Autodesk Fusion 360 part; units mm, degrees
(part 3 of 6)
  line L1808 (236.2761, -16.388) -> (236.2761, -22.338)
  line L1809 (236.2761, -22.338) -> (235.476, -22.338)
  line L1810 (235.476, -22.338) -> (235.476, -25.288)
  line L1811 (235.476, -25.288) -> (236.2761, -25.288)
  line L1812 (236.2761, -25.288) -> (236.2761, -26.288)
  line L1813 (236.2761, -26.288) -> (250.126, -26.288)
  line L1814 (250.126, -26.288) -> (250.126, -25.288)
  line L1815 (250.126, -25.288) -> (250.9261, -25.288)
  line L1816 (250.9261, -25.288) -> (250.9261, -22.338)
  line L1817 (250.9261, -22.338) -> (250.126, -22.338)
  line L1818 (250.126, -22.338) -> (250.126, -16.388)
  line L1819 (250.126, -16.388) -> (250.9261, -16.388)
  line L1820 (250.9261, -16.388) -> (250.9261, -13.438)
  line L1821 (250.9261, -13.438) -> (250.126, -13.438)
  line L1822 (250.126, -13.438) -> (250.126, -12.438)
  line L1823 (250.126, -12.438) -> (236.2761, -12.438)
  line L1824 (255.3261, -12.438) -> (255.3261, -13.438)
  line L1825 (255.3261, -13.438) -> (254.526, -13.438)
  line L1826 (254.526, -13.438) -> (254.526, -16.388)
  line L1827 (254.526, -16.388) -> (255.3261, -16.388)
  line L1828 (255.3261, -16.388) -> (255.3261, -22.338)
  line L1829 (255.3261, -22.338) -> (254.526, -22.338)
  line L1830 (254.526, -22.338) -> (254.526, -25.288)
  line L1831 (254.526, -25.288) -> (255.3261, -25.288)
  line L1832 (255.3261, -25.288) -> (255.3261, -26.288)
  line L1833 (255.3261, -26.288) -> (269.1765, -26.288)
  line L1834 (269.1765, -26.288) -> (269.1765, -25.288)
  line L1835 (269.1765, -25.288) -> (269.9755, -25.288)
  line L1836 (269.9755, -25.288) -> (269.9755, -22.338)
  line L1837 (269.9755, -22.338) -> (269.1765, -22.338)
  line L1838 (269.1765, -22.338) -> (269.1765, -16.388)
  line L1839 (269.1765, -16.388) -> (269.9755, -16.388)
  line L1840 (269.9755, -16.388) -> (269.9755, -13.438)
  line L1841 (269.9755, -13.438) -> (269.1765, -13.438)
  line L1842 (269.1765, -13.438) -> (269.1765, -12.438)
  line L1843 (269.1765, -12.438) -> (255.3261, -12.438)
extrude "Extrude1" add sketch "Sketch3" along normal blind 1.5 makes body 1
sketch "sketch 18250" plane through (138.5014, -57.3885, -4) normal (0, 0, 1) x (-1, 0, 0)
  line L0 (-186.1132, -52.3735) -> (-185.7375, -52.3875)
  line L1 (-185.7375, -52.3875) -> (128.5877, -52.3885)
  line L2 (128.5877, -52.3885) -> (128.9617, -52.3735)
  line L3 (128.9617, -52.3735) -> (129.3327, -52.3295)
  line L4 (129.3327, -52.3295) -> (129.6997, -52.2565)
  line L5 (129.6997, -52.2565) -> (130.0597, -52.1545)
  line L6 (130.0597, -52.1545) -> (130.4107, -52.0255)
  line L7 (130.4107, -52.0255) -> (130.7497, -51.8685)
  line L8 (130.7497, -51.8685) -> (131.0757, -51.6865)
  line L9 (131.0757, -51.6865) -> (131.3867, -51.4785)
  line L10 (131.3867, -51.4785) -> (131.6807, -51.2465)
  line L11 (131.6807, -51.2465) -> (131.9557, -50.9935)
  line L12 (131.9557, -50.9935) -> (132.2087, -50.7185)
  line L13 (132.2087, -50.7185) -> (132.4407, -50.4245)
  line L14 (132.4407, -50.4245) -> (132.6487, -50.1135)
  line L15 (132.6487, -50.1135) -> (132.8307, -49.7875)
  line L16 (132.8307, -49.7875) -> (132.9877, -49.4485)
  line L17 (132.9877, -49.4485) -> (133.1167, -49.0975)
  line L18 (133.1167, -49.0975) -> (133.2187, -48.7375)
  line L19 (133.2187, -48.7375) -> (133.2917, -48.3705)
  line L20 (133.2917, -48.3705) -> (133.3357, -47.9995)
  line L21 (133.3357, -47.9995) -> (133.3497, -47.6255)
  line L22 (133.3497, -47.6255) -> (133.3507, 76.2005)
  line L23 (133.3507, 76.2005) -> (133.3357, 76.5744)
  line L24 (133.3357, 76.5744) -> (133.2917, 76.9456)
  line L25 (133.2917, 76.9456) -> (133.2187, 77.3126)
  line L26 (133.2187, 77.3126) -> (133.1167, 77.6724)
  line L27 (133.1167, 77.6724) -> (132.9877, 78.0235)
  line L28 (132.9877, 78.0235) -> (132.8307, 78.3625)
  line L29 (132.8307, 78.3625) -> (132.6487, 78.6884)
  line L30 (132.6487, 78.6884) -> (132.4407, 78.9996)
  line L31 (132.4407, 78.9996) -> (132.2087, 79.2935)
  line L32 (132.2087, 79.2935) -> (131.9557, 79.5684)
  line L33 (131.9557, 79.5684) -> (131.6807, 79.8216)
  line L34 (131.6807, 79.8216) -> (131.3867, 80.0534)
  line L35 (131.3867, 80.0534) -> (131.0757, 80.2614)
  line L36 (131.0757, 80.2614) -> (130.7497, 80.4434)
  line L37 (130.7497, 80.4434) -> (130.4107, 80.6006)
  line L38 (130.4107, 80.6006) -> (130.0597, 80.7294)
  line L39 (130.0597, 80.7294) -> (129.6997, 80.8316)
  line L40 (129.6997, 80.8316) -> (129.3327, 80.9046)
  line L41 (129.3327, 80.9046) -> (128.9617, 80.9485)
  line L42 (128.9617, 80.9485) -> (128.5877, 80.9636)
  line L43 (128.5877, 80.9636) -> (-185.7375, 80.9636)
  line L44 (-185.7375, 80.9636) -> (-186.1132, 80.9485)
  line L45 (-186.1132, 80.9485) -> (-186.4836, 80.9046)
  line L46 (-186.4836, 80.9046) -> (-186.8514, 80.8316)
  line L47 (-186.8514, 80.8316) -> (-187.2112, 80.7294)
  line L48 (-187.2112, 80.7294) -> (-187.5605, 80.6006)
  line L49 (-187.5605, 80.6006) -> (-187.8992, 80.4434)
  line L50 (-187.8992, 80.4434) -> (-188.2272, 80.2614)
  line L51 (-188.2272, 80.2614) -> (-188.5368, 80.0534)
  line L52 (-188.5368, 80.0534) -> (-188.8305, 79.8216)
  line L53 (-188.8305, 79.8216) -> (-189.1057, 79.5684)
  line L54 (-189.1057, 79.5684) -> (-189.3597, 79.2935)
  line L55 (-189.3597, 79.2935) -> (-189.5925, 78.9996)
  line L56 (-189.5925, 78.9996) -> (-189.7989, 78.6884)
  line L57 (-189.7989, 78.6884) -> (-189.9814, 78.3625)
  line L58 (-189.9814, 78.3625) -> (-190.1375, 78.0235)
  line L59 (-190.1375, 78.0235) -> (-190.2672, 77.6724)
  line L60 (-190.2672, 77.6724) -> (-190.3704, 77.3126)
  line L61 (-190.3704, 77.3126) -> (-190.4418, 76.9456)
  line L62 (-190.4418, 76.9456) -> (-190.4868, 76.5744)
  line L63 (-190.4868, 76.5744) -> (-190.5, 76.2005)
  line L64 (-190.5, 76.2005) -> (-190.5, -47.6255)
  line L65 (-190.5, -47.6255) -> (-190.4868, -47.9995)
  line L66 (-190.4868, -47.9995) -> (-190.4418, -48.3705)
  line L67 (-190.4418, -48.3705) -> (-190.3704, -48.7375)
  line L68 (-190.3704, -48.7375) -> (-190.2672, -49.0975)
  line L69 (-190.2672, -49.0975) -> (-190.1375, -49.4485)
  line L70 (-190.1375, -49.4485) -> (-189.9814, -49.7875)
  line L71 (-189.9814, -49.7875) -> (-189.7989, -50.1135)
  line L72 (-189.7989, -50.1135) -> (-189.5925, -50.4245)
  line L73 (-189.5925, -50.4245) -> (-189.3597, -50.7185)
  line L74 (-189.3597, -50.7185) -> (-189.1057, -50.9935)
  line L75 (-189.1057, -50.9935) -> (-188.8305, -51.2465)
  line L76 (-188.8305, -51.2465) -> (-188.5368, -51.4785)
  line L77 (-188.5368, -51.4785) -> (-188.2272, -51.6865)
  line L78 (-188.2272, -51.6865) -> (-187.8992, -51.8685)
  line L79 (-187.8992, -51.8685) -> (-187.5605, -52.0255)
  line L80 (-187.5605, -52.0255) -> (-187.2112, -52.1545)
  line L81 (-187.2112, -52.1545) -> (-186.8514, -52.2565)
  line L82 (-186.8514, -52.2565) -> (-186.4836, -52.3295)
  line L83 (-186.4836, -52.3295) -> (-186.1132, -52.3735)
  circle A0 centre (128.5875, 76.2) radius 1.1
  arc A1 (117.7379, 65.4486) -> (118.4252, 66.1358) centre (117.9984, 65.8753) ccw
  arc A2 (117.7379, 65.4486) -> (117.5816, 65.4925) centre (117.5817, 65.1928) ccw
  line L84 (117.5816, 65.4925) -> (116.6813, 65.4925)
  line L85 (116.6813, 65.4925) -> (115.7809, 65.4925)
  arc A3 (115.7809, 65.4925) -> (115.6246, 65.4486) centre (115.7809, 65.1925) ccw
  arc A4 (114.9373, 66.1358) -> (115.6246, 65.4486) centre (115.3641, 65.8753) ccw
  arc A5 (114.9373, 66.1358) -> (114.9812, 66.2921) centre (114.6813, 66.2921) ccw
  line L86 (114.9812, 66.2921) -> (114.9813, 66.9925)
  line L87 (114.9813, 66.9925) -> (114.9813, 67.6929)
  arc A6 (114.9813, 67.6929) -> (114.9373, 67.8492) centre (114.6813, 67.6929) ccw
  arc A7 (115.6246, 68.5364) -> (114.9373, 67.8492) centre (115.3641, 68.1097) ccw
  arc A8 (115.6246, 68.5364) -> (115.7809, 68.4925) centre (115.7809, 68.7925) ccw
  line L88 (115.7809, 68.4925) -> (116.6813, 68.4925)
  line L89 (116.6813, 68.4925) -> (117.5816, 68.4925)
  arc A9 (117.5816, 68.4925) -> (117.7379, 68.5364) centre (117.5816, 68.7925) ccw
  arc A10 (118.4252, 67.8492) -> (117.7379, 68.5364) centre (117.9984, 68.1097) ccw
  arc A11 (118.4252, 67.8492) -> (118.3812, 67.6929) centre (118.6813, 67.6928) ccw
  line L90 (118.3812, 67.6929) -> (118.3812, 66.9925)
  line L91 (118.3812, 66.9925) -> (118.3812, 66.2921)
  arc A12 (118.3812, 66.2921) -> (118.4252, 66.1358) centre (118.6813, 66.2922) ccw
  circle A13 centre (121.7613, 61.9125) radius 0.875
  circle A14 centre (116.6813, 61.9125) radius 1.9939
  circle A15 centre (111.6013, 61.9125) radius 0.875
  arc A16 (93.9254, 65.4486) -> (94.6127, 66.1358) centre (94.1859, 65.8753) ccw
  arc A17 (93.9254, 65.4486) -> (93.7691, 65.4925) centre (93.7692, 65.1928) ccw
  line L92 (93.7691, 65.4925) -> (92.8688, 65.4925)
  line L93 (92.8688, 65.4925) -> (91.9684, 65.4925)
  arc A18 (91.9684, 65.4925) -> (91.8121, 65.4486) centre (91.9684, 65.1925) ccw
  arc A19 (91.1248, 66.1358) -> (91.8121, 65.4486) centre (91.5516, 65.8753) ccw
  arc A20 (91.1248, 66.1358) -> (91.1687, 66.2921) centre (90.8688, 66.2921) ccw
  line L94 (91.1687, 66.2921) -> (91.1688, 66.9925)
  line L95 (91.1688, 66.9925) -> (91.1688, 67.6929)
  arc A21 (91.1688, 67.6929) -> (91.1248, 67.8492) centre (90.8688, 67.6929) ccw
  arc A22 (91.8121, 68.5364) -> (91.1248, 67.8492) centre (91.5516, 68.1097) ccw
  arc A23 (91.8121, 68.5364) -> (91.9684, 68.4925) centre (91.9684, 68.7925) ccw
  line L96 (91.9684, 68.4925) -> (92.8688, 68.4925)
  line L97 (92.8688, 68.4925) -> (93.7691, 68.4925)
  arc A24 (93.7691, 68.4925) -> (93.9254, 68.5364) centre (93.7691, 68.7925) ccw
  arc A25 (94.6127, 67.8492) -> (93.9254, 68.5364) centre (94.1859, 68.1097) ccw
  arc A26 (94.6127, 67.8492) -> (94.5687, 67.6929) centre (94.8688, 67.6928) ccw
  line L98 (94.5687, 67.6929) -> (94.5687, 66.9925)
  line L99 (94.5687, 66.9925) -> (94.5687, 66.2921)
  arc A27 (94.5687, 66.2921) -> (94.6127, 66.1358) centre (94.8688, 66.2922) ccw
  circle A28 centre (97.9488, 61.9125) radius 0.875
  circle A29 centre (92.8688, 61.9125) radius 1.9939
  circle A30 centre (87.7887, 61.9125) radius 0.875
  circle A31 centre (74.1363, 61.9125) radius 0.875
  arc A32 (70.1129, 65.4486) -> (70.8002, 66.1358) centre (70.3734, 65.8753) ccw
  arc A33 (70.1129, 65.4486) -> (69.9566, 65.4925) centre (69.9567, 65.1928) ccw
  line L100 (69.9566, 65.4925) -> (69.0563, 65.4925)
  line L101 (69.0563, 65.4925) -> (68.1559, 65.4925)
  arc A34 (68.1559, 65.4925) -> (67.9996, 65.4486) centre (68.1559, 65.1925) ccw
  arc A35 (67.3123, 66.1358) -> (67.9996, 65.4486) centre (67.7391, 65.8753) ccw
  arc A36 (67.3123, 66.1358) -> (67.3562, 66.2921) centre (67.0563, 66.2921) ccw
  line L102 (67.3562, 66.2921) -> (67.3563, 66.9925)
  line L103 (67.3563, 66.9925) -> (67.3563, 67.6929)
  arc A37 (67.3563, 67.6929) -> (67.3123, 67.8492) centre (67.0563, 67.6929) ccw
  arc A38 (67.9996, 68.5364) -> (67.3123, 67.8492) centre (67.7391, 68.1097) ccw
  arc A39 (67.9996, 68.5364) -> (68.1559, 68.4925) centre (68.1559, 68.7925) ccw
  line L104 (68.1559, 68.4925) -> (69.0563, 68.4925)
  line L105 (69.0563, 68.4925) -> (69.9566, 68.4925)
  arc A40 (69.9566, 68.4925) -> (70.1129, 68.5364) centre (69.9566, 68.7925) ccw
  arc A41 (70.8002, 67.8492) -> (70.1129, 68.5364) centre (70.3734, 68.1097) ccw
  arc A42 (70.8002, 67.8492) -> (70.7562, 67.6929) centre (71.0563, 67.6928) ccw
  line L106 (70.7562, 67.6929) -> (70.7562, 66.9925)
  line L107 (70.7562, 66.9925) -> (70.7562, 66.2921)
  arc A43 (70.7562, 66.2921) -> (70.8002, 66.1358) centre (71.0563, 66.2922) ccw
  circle A44 centre (69.0563, 61.9125) radius 1.9939
  circle A45 centre (63.9763, 61.9125) radius 0.875
  circle A46 centre (120.4913, 59.3725) radius 1.5
  circle A47 centre (114.1412, 56.8325) radius 1.5
  circle A48 centre (96.6788, 59.3725) radius 1.5
  circle A49 centre (90.3288, 56.8325) radius 1.5
  arc A50 (108.2129, 46.3986) -> (108.9002, 47.0858) centre (108.4734, 46.8253) ccw
  arc A51 (108.2129, 46.3986) -> (108.0566, 46.4425) centre (108.0567, 46.1428) ccw
  line L108 (108.0566, 46.4425) -> (107.1563, 46.4425)
  line L109 (107.1563, 46.4425) -> (106.2559, 46.4425)
  arc A52 (106.2559, 46.4425) -> (106.0996, 46.3986) centre (106.2559, 46.1425) ccw
  arc A53 (105.4123, 47.0858) -> (106.0996, 46.3986) centre (105.8391, 46.8253) ccw
  arc A54 (105.4123, 47.0858) -> (105.4562, 47.2421) centre (105.1563, 47.2421) ccw
  line L110 (105.4562, 47.2421) -> (105.4563, 47.9425)
  line L111 (105.4563, 47.9425) -> (105.4563, 48.6429)
  arc A55 (105.4563, 48.6429) -> (105.4123, 48.7992) centre (105.1563, 48.6429) ccw
  arc A56 (106.0996, 49.4864) -> (105.4123, 48.7992) centre (105.8391, 49.0597) ccw
  arc A57 (106.0996, 49.4864) -> (106.2559, 49.4425) centre (106.2559, 49.7425) ccw
  line L112 (106.2559, 49.4425) -> (107.1562, 49.4425)
  line L113 (107.1563, 49.4425) -> (108.0566, 49.4425)
  arc A58 (108.0566, 49.4425) -> (108.2129, 49.4864) centre (108.0566, 49.7425) ccw
  arc A59 (108.9002, 48.7992) -> (108.2129, 49.4864) centre (108.4734, 49.0597) ccw
  arc A60 (108.9002, 48.7992) -> (108.8562, 48.6429) centre (109.1563, 48.6428) ccw
  line L114 (108.8562, 48.6429) -> (108.8563, 47.9425)
  line L115 (108.8563, 47.9425) -> (108.8563, 47.2421)
  arc A61 (108.8563, 47.2421) -> (108.9002, 47.0858) centre (109.1563, 47.2422) ccw
  circle A62 centre (72.8662, 59.3725) radius 1.5
  circle A63 centre (66.5162, 56.8325) radius 1.5
  arc A64 (77.2567, 46.3986) -> (77.9439, 47.0858) centre (77.5172, 46.8253) ccw
  arc A65 (77.2567, 46.3986) -> (77.1004, 46.4425) centre (77.1004, 46.1428) ccw
  line L116 (77.1004, 46.4425) -> (76.2, 46.4425)
  line L117 (76.2, 46.4425) -> (75.2996, 46.4425)
  arc A66 (75.2996, 46.4425) -> (75.1433, 46.3986) centre (75.2996, 46.1425) ccw
  arc A67 (74.4561, 47.0858) -> (75.1433, 46.3986) centre (74.8828, 46.8253) ccw
  arc A68 (74.4561, 47.0858) -> (74.5, 47.2421) centre (74.2, 47.2421) ccw
  line L118 (74.5, 47.2421) -> (74.5, 47.9425)
  line L119 (74.5, 47.9425) -> (74.5, 48.6429)
  arc A69 (74.5, 48.6429) -> (74.4561, 48.7992) centre (74.2, 48.6429) ccw
  arc A70 (75.1433, 49.4864) -> (74.4561, 48.7992) centre (74.8828, 49.0597) ccw
  arc A71 (75.1433, 49.4864) -> (75.2996, 49.4425) centre (75.2996, 49.7425) ccw
  line L120 (75.2996, 49.4425) -> (76.2, 49.4425)
  line L121 (76.2, 49.4425) -> (77.1004, 49.4425)
  arc A72 (77.1004, 49.4425) -> (77.2567, 49.4864) centre (77.1003, 49.7425) ccw
  arc A73 (77.9439, 48.7992) -> (77.2567, 49.4864) centre (77.5172, 49.0597) ccw
  arc A74 (77.9439, 48.7992) -> (77.9, 48.6429) centre (78.2001, 48.6428) ccw
  line L122 (77.9, 48.6429) -> (77.9, 47.9425)
  line L123 (77.9, 47.9425) -> (77.9, 47.2421)
  arc A75 (77.9, 47.2421) -> (77.9439, 47.0858) centre (78.2, 47.2422) ccw
  arc A76 (58.2067, 46.3986) -> (58.8939, 47.0858) centre (58.4672, 46.8253) ccw
  arc A77 (58.2067, 46.3986) -> (58.0504, 46.4425) centre (58.0504, 46.1428) ccw
  line L124 (58.0504, 46.4425) -> (57.15, 46.4425)
  line L125 (57.15, 46.4425) -> (56.2496, 46.4425)
  arc A78 (56.2496, 46.4425) -> (56.0933, 46.3986) centre (56.2496, 46.1425) ccw
  arc A79 (55.4061, 47.0858) -> (56.0933, 46.3986) centre (55.8328, 46.8253) ccw
  arc A80 (55.4061, 47.0858) -> (55.45, 47.2421) centre (55.15, 47.2421) ccw
  line L126 (55.45, 47.2421) -> (55.45, 47.9425)
  line L127 (55.45, 47.9425) -> (55.45, 48.6429)
  arc A81 (55.45, 48.6429) -> (55.4061, 48.7992) centre (55.15, 48.6429) ccw
  arc A82 (56.0933, 49.4864) -> (55.4061, 48.7992) centre (55.8328, 49.0597) ccw
  arc A83 (56.0933, 49.4864) -> (56.2496, 49.4425) centre (56.2496, 49.7425) ccw
  line L128 (56.2496, 49.4425) -> (57.15, 49.4425)
  line L129 (57.15, 49.4425) -> (58.0504, 49.4425)
  arc A84 (58.0504, 49.4425) -> (58.2067, 49.4864) centre (58.0503, 49.7425) ccw
  arc A85 (58.8939, 48.7992) -> (58.2067, 49.4864) centre (58.4672, 49.0597) ccw
  arc A86 (58.8939, 48.7992) -> (58.85, 48.6429) centre (59.1501, 48.6428) ccw
  line L130 (58.85, 48.6429) -> (58.85, 47.9425)
  line L131 (58.85, 47.9425) -> (58.85, 47.2421)
  arc A87 (58.85, 47.2421) -> (58.8939, 47.0858) centre (59.15, 47.2422) ccw
  circle A88 centre (30.9563, 76.2) radius 1.1
  arc A89 (-4.1252, 66.1358) -> (-3.4379, 65.4486) centre (-3.6984, 65.8753) ccw
  arc A90 (-4.1252, 66.1358) -> (-4.0813, 66.2921) centre (-4.3812, 66.2921) ccw
  line L132 (-4.0812, 66.2921) -> (-4.0812, 66.9925)
  line L133 (-4.0812, 66.9925) -> (-4.0812, 67.6929)
  arc A91 (-4.0812, 67.6929) -> (-4.1252, 67.8492) centre (-4.3812, 67.6929) ccw
  arc A92 (-3.4379, 68.5364) -> (-4.1252, 67.8492) centre (-3.6984, 68.1097) ccw
  arc A93 (-3.4379, 68.5364) -> (-3.2816, 68.4925) centre (-3.2816, 68.7925) ccw
  line L134 (-3.2816, 68.4925) -> (-2.3813, 68.4925)
  line L135 (-2.3813, 68.4925) -> (-1.4809, 68.4925)
  arc A94 (-1.4809, 68.4925) -> (-1.3246, 68.5364) centre (-1.4809, 68.7925) ccw
  arc A95 (-0.6373, 67.8492) -> (-1.3246, 68.5364) centre (-1.0641, 68.1097) ccw
  arc A96 (-0.6373, 67.8492) -> (-0.6813, 67.6929) centre (-0.3812, 67.6928) ccw
  line L136 (-0.6812, 67.6929) -> (-0.6813, 66.9925)
  line L137 (-0.6813, 66.9925) -> (-0.6813, 66.2921)
  arc A97 (-0.6813, 66.2921) -> (-0.6373, 66.1358) centre (-0.3812, 66.2922) ccw
  arc A98 (-1.3246, 65.4486) -> (-0.6373, 66.1358) centre (-1.0641, 65.8753) ccw
  arc A99 (-1.3246, 65.4486) -> (-1.4809, 65.4925) centre (-1.4808, 65.1928) ccw
  line L138 (-1.4809, 65.4925) -> (-2.3813, 65.4925)
  line L139 (-2.3813, 65.4925) -> (-3.2816, 65.4925)
  arc A100 (-3.2816, 65.4925) -> (-3.4379, 65.4486) centre (-3.2816, 65.1925) ccw
  circle A101 centre (2.6988, 61.9125) radius 0.875
  circle A102 centre (-2.3813, 61.9125) radius 1.9939
  circle A103 centre (-7.4613, 61.9125) radius 0.875
  arc A104 (39.1567, 46.3986) -> (39.8439, 47.0858) centre (39.4172, 46.8253) ccw
  arc A105 (39.1567, 46.3986) -> (39.0004, 46.4425) centre (39.0004, 46.1428) ccw
  line L140 (39.0004, 46.4425) -> (38.1, 46.4425)
  line L141 (38.1, 46.4425) -> (37.1996, 46.4425)
  arc A106 (37.1996, 46.4425) -> (37.0433, 46.3986) centre (37.1996, 46.1425) ccw
  arc A107 (36.3561, 47.0858) -> (37.0433, 46.3986) centre (36.7828, 46.8253) ccw
  arc A108 (36.3561, 47.0858) -> (36.4, 47.2421) centre (36.1, 47.2421) ccw
  line L142 (36.4, 47.2421) -> (36.4, 47.9425)
  line L143 (36.4, 47.9425) -> (36.4, 48.6429)
  arc A109 (36.4, 48.6429) -> (36.3561, 48.7992) centre (36.1, 48.6429) ccw
  arc A110 (37.0433, 49.4864) -> (36.3561, 48.7992) centre (36.7828, 49.0597) ccw
  arc A111 (37.0433, 49.4864) -> (37.1996, 49.4425) centre (37.1996, 49.7425) ccw
  line L144 (37.1996, 49.4425) -> (38.1, 49.4425)
  line L145 (38.1, 49.4425) -> (39.0004, 49.4425)
  arc A112 (39.0004, 49.4425) -> (39.1567, 49.4864) centre (39.0003, 49.7425) ccw
  arc A113 (39.8439, 48.7992) -> (39.1567, 49.4864) centre (39.4172, 49.0597) ccw
  arc A114 (39.8439, 48.7992) -> (39.8, 48.6429) centre (40.1001, 48.6428) ccw
  line L146 (39.8, 48.6429) -> (39.8, 47.9425)
  line L147 (39.8, 47.9425) -> (39.8, 47.2421)
  arc A115 (39.8, 47.2421) -> (39.8439, 47.0858) centre (40.1, 47.2422) ccw
  arc A116 (20.1067, 46.3986) -> (20.7939, 47.0858) centre (20.3672, 46.8253) ccw
  arc A117 (20.1067, 46.3986) -> (19.9504, 46.4425) centre (19.9504, 46.1428) ccw
  line L148 (19.9504, 46.4425) -> (19.05, 46.4425)
  line L149 (19.05, 46.4425) -> (18.1496, 46.4425)
  arc A118 (18.1496, 46.4425) -> (17.9933, 46.3986) centre (18.1496, 46.1425) ccw
  arc A119 (17.3061, 47.0858) -> (17.9933, 46.3986) centre (17.7328, 46.8253) ccw
  arc A120 (17.3061, 47.0858) -> (17.35, 47.2421) centre (17.05, 47.2421) ccw
  line L150 (17.35, 47.2421) -> (17.35, 47.9425)
  line L151 (17.35, 47.9425) -> (17.35, 48.6429)
  arc A121 (17.35, 48.6429) -> (17.3061, 48.7992) centre (17.05, 48.6429) ccw
  arc A122 (17.9933, 49.4864) -> (17.3061, 48.7992) centre (17.7328, 49.0597) ccw
  arc A123 (17.9933, 49.4864) -> (18.1496, 49.4425) centre (18.1496, 49.7425) ccw
  line L152 (18.1496, 49.4425) -> (19.05, 49.4425)
  line L153 (19.05, 49.4425) -> (19.9504, 49.4425)
  arc A124 (19.9504, 49.4425) -> (20.1067, 49.4864) centre (19.9503, 49.7425) ccw
  arc A125 (20.7939, 48.7992) -> (20.1067, 49.4864) centre (20.3672, 49.0597) ccw
  arc A126 (20.7939, 48.7992) -> (20.75, 48.6429) centre (21.0501, 48.6428) ccw
  line L154 (20.75, 48.6429) -> (20.75, 47.9425)
  line L155 (20.75, 47.9425) -> (20.75, 47.2421)
  arc A127 (20.75, 47.2421) -> (20.7939, 47.0858) centre (21.05, 47.2422) ccw
  circle A128 centre (1.4287, 59.3725) radius 1.5
  circle A129 centre (-4.9212, 56.8325) radius 1.5
  arc A130 (1.0567, 46.3986) -> (1.7439, 47.0858) centre (1.3172, 46.8253) ccw
  arc A131 (1.0567, 46.3986) -> (0.9004, 46.4425) centre (0.9004, 46.1428) ccw
  line L156 (0.9004, 46.4425) -> (0, 46.4425)
  line L157 (0, 46.4425) -> (-0.9004, 46.4425)
  arc A132 (-0.9004, 46.4425) -> (-1.0567, 46.3986) centre (-0.9004, 46.1425) ccw
  arc A133 (-1.7439, 47.0858) -> (-1.0567, 46.3986) centre (-1.3172, 46.8253) ccw
  arc A134 (-1.7439, 47.0858) -> (-1.7, 47.2421) centre (-2, 47.2421) ccw
  line L158 (-1.7, 47.2421) -> (-1.7, 47.9425)
  line L159 (-1.7, 47.9425) -> (-1.7, 48.6429)
  arc A135 (-1.7, 48.6429) -> (-1.7439, 48.7992) centre (-2, 48.6429) ccw
  arc A136 (-1.0567, 49.4864) -> (-1.7439, 48.7992) centre (-1.3172, 49.0597) ccw
  arc A137 (-1.0567, 49.4864) -> (-0.9004, 49.4425) centre (-0.9004, 49.7425) ccw
  line L160 (-0.9004, 49.4425) -> (0, 49.4425)
  line L161 (0, 49.4425) -> (0.9004, 49.4425)
  arc A138 (0.9004, 49.4425) -> (1.0567, 49.4864) centre (0.9003, 49.7425) ccw
  arc A139 (1.7439, 48.7992) -> (1.0567, 49.4864) centre (1.3172, 49.0597) ccw
  arc A140 (1.7439, 48.7992) -> (1.7, 48.6429) centre (2.0001, 48.6428) ccw
  line L162 (1.7, 48.6429) -> (1.7, 47.9425)
  line L163 (1.7, 47.9425) -> (1.7, 47.2421)
  arc A141 (1.7, 47.2421) -> (1.7439, 47.0858) centre (2, 47.2422) ccw
  arc A142 (-20.7939, 47.0858) -> (-20.1067, 46.3986) centre (-20.3672, 46.8253) ccw
  arc A143 (-20.7939, 47.0858) -> (-20.75, 47.2421) centre (-21.05, 47.2421) ccw
  line L164 (-20.75, 47.2421) -> (-20.75, 47.9425)
  line L165 (-20.75, 47.9425) -> (-20.75, 48.6429)
  arc A144 (-20.75, 48.6429) -> (-20.7939, 48.7992) centre (-21.05, 48.6429) ccw
  arc A145 (-20.1067, 49.4864) -> (-20.7939, 48.7992) centre (-20.3672, 49.0597) ccw
  arc A146 (-20.1067, 49.4864) -> (-19.9504, 49.4425) centre (-19.9504, 49.7425) ccw
  line L166 (-19.9504, 49.4425) -> (-19.05, 49.4425)
  line L167 (-19.05, 49.4425) -> (-18.1496, 49.4425)
  arc A147 (-18.1496, 49.4425) -> (-17.9933, 49.4864) centre (-18.1497, 49.7425) ccw
  arc A148 (-17.3061, 48.7992) -> (-17.9933, 49.4864) centre (-17.7328, 49.0597) ccw
  arc A149 (-17.3061, 48.7992) -> (-17.35, 48.6429) centre (-17.0499, 48.6428) ccw
  line L168 (-17.35, 48.6429) -> (-17.35, 47.9425)
  line L169 (-17.35, 47.9425) -> (-17.35, 47.2421)
  arc A150 (-17.35, 47.2421) -> (-17.3061, 47.0858) centre (-17.05, 47.2422) ccw
  arc A151 (-17.9933, 46.3986) -> (-17.3061, 47.0858) centre (-17.7328, 46.8253) ccw
  arc A152 (-17.9933, 46.3986) -> (-18.1496, 46.4425) centre (-18.1496, 46.1428) ccw
  line L170 (-18.1496, 46.4425) -> (-19.05, 46.4425)
  line L171 (-19.05, 46.4425) -> (-19.9504, 46.4425)
  arc A153 (-19.9504, 46.4425) -> (-20.1067, 46.3986) centre (-19.9504, 46.1425) ccw
  circle A154 centre (112.2362, 42.8625) radius 0.875
  circle A155 centre (110.9663, 40.3225) radius 1.5
  circle A156 centre (107.1563, 42.8625) radius 1.9939
  circle A157 centre (102.0763, 42.8625) radius 0.875
  circle A158 centre (104.6162, 37.7825) radius 1.5
  circle A159 centre (81.28, 42.8625) radius 0.875
  circle A160 centre (76.2, 42.8625) radius 1.9939
  circle A161 centre (71.12, 42.8625) radius 0.875
  circle A162 centre (80.01, 40.3225) radius 1.5
  circle A163 centre (73.66, 37.7825) radius 1.5
  circle A164 centre (62.23, 42.8625) radius 0.875
  circle A165 centre (57.15, 42.8625) radius 1.9939
  circle A166 centre (52.07, 42.8625) radius 0.875
  circle A167 centre (60.96, 40.3225) radius 1.5
  circle A168 centre (54.61, 37.7825) radius 1.5
  arc A169 (112.9754, 27.3486) -> (113.6627, 28.0358) centre (113.2359, 27.7753) ccw
  arc A170 (112.9754, 27.3486) -> (112.8191, 27.3925) centre (112.8192, 27.0928) ccw
  line L172 (112.8191, 27.3925) -> (111.9188, 27.3925)
  line L173 (111.9188, 27.3925) -> (111.0184, 27.3925)
  arc A171 (111.0184, 27.3925) -> (110.8621, 27.3486) centre (111.0184, 27.0925) ccw
  arc A172 (110.1748, 28.0358) -> (110.8621, 27.3486) centre (110.6016, 27.7753) ccw
  arc A173 (110.1748, 28.0358) -> (110.2187, 28.1921) centre (109.9188, 28.1921) ccw
  line L174 (110.2187, 28.1921) -> (110.2188, 28.8925)
  line L175 (110.2188, 28.8925) -> (110.2188, 29.5929)
  arc A174 (110.2188, 29.5929) -> (110.1748, 29.7492) centre (109.9188, 29.5929) ccw
  arc A175 (110.8621, 30.4364) -> (110.1748, 29.7492) centre (110.6016, 30.0097) ccw
  arc A176 (110.8621, 30.4364) -> (111.0184, 30.3925) centre (111.0184, 30.6925) ccw
  line L176 (111.0184, 30.3925) -> (111.9188, 30.3925)
  line L177 (111.9188, 30.3925) -> (112.8191, 30.3925)
  arc A177 (112.8191, 30.3925) -> (112.9754, 30.4364) centre (112.8191, 30.6925) ccw
  arc A178 (113.6627, 29.7492) -> (112.9754, 30.4364) centre (113.2359, 30.0097) ccw
  arc A179 (113.6627, 29.7492) -> (113.6187, 29.5929) centre (113.9188, 29.5928) ccw
  line L178 (113.6187, 29.5929) -> (113.6188, 28.8925)
  line L179 (113.6188, 28.8925) -> (113.6188, 28.1921)
  arc A180 (113.6188, 28.1921) -> (113.6627, 28.0358) centre (113.9188, 28.1922) ccw
  circle A181 centre (116.9988, 23.8125) radius 0.875
  circle A182 centre (111.9188, 23.8125) radius 1.9939
  circle A183 centre (106.8388, 23.8125) radius 0.875
  circle A184 centre (90.805, 23.8125) radius 0.875
  circle A185 centre (115.7288, 21.2725) radius 1.5
  circle A186 centre (128.5875, 14.2875) radius 1.1
  circle A187 centre (109.3787, 18.7325) radius 1.5
  arc A188 (86.7817, 27.3486) -> (87.4689, 28.0358) centre (87.0422, 27.7753) ccw
  arc A189 (86.7817, 27.3486) -> (86.6254, 27.3925) centre (86.6254, 27.0928) ccw
  line L180 (86.6254, 27.3925) -> (85.725, 27.3925)
  line L181 (85.725, 27.3925) -> (84.8246, 27.3925)
  arc A190 (84.8246, 27.3925) -> (84.6683, 27.3486) centre (84.8246, 27.0925) ccw
  arc A191 (83.9811, 28.0358) -> (84.6683, 27.3486) centre (84.4078, 27.7753) ccw
  arc A192 (83.9811, 28.0358) -> (84.025, 28.1921) centre (83.725, 28.1921) ccw
  line L182 (84.025, 28.1921) -> (84.025, 28.8925)
  line L183 (84.025, 28.8925) -> (84.025, 29.5929)
  arc A193 (84.025, 29.5929) -> (83.9811, 29.7492) centre (83.725, 29.5929) ccw
  arc A194 (84.6683, 30.4364) -> (83.9811, 29.7492) centre (84.4078, 30.0097) ccw
  arc A195 (84.6683, 30.4364) -> (84.8246, 30.3925) centre (84.8246, 30.6925) ccw
  line L184 (84.8246, 30.3925) -> (85.725, 30.3925)
  line L185 (85.725, 30.3925) -> (86.6254, 30.3925)
  arc A196 (86.6254, 30.3925) -> (86.7817, 30.4364) centre (86.6253, 30.6925) ccw
  arc A197 (87.4689, 29.7492) -> (86.7817, 30.4364) centre (87.0422, 30.0097) ccw
  arc A198 (87.4689, 29.7492) -> (87.425, 29.5929) centre (87.7251, 29.5928) ccw
  line L186 (87.425, 29.5929) -> (87.425, 28.8925)
  line L187 (87.425, 28.8925) -> (87.425, 28.1921)
  arc A199 (87.425, 28.1921) -> (87.4689, 28.0358) centre (87.725, 28.1922) ccw
  circle A200 centre (85.725, 23.8125) radius 1.9939
  circle A201 centre (80.645, 23.8125) radius 0.875
  circle A202 centre (71.755, 23.8125) radius 0.875
  arc A203 (67.7317, 27.3486) -> (68.4189, 28.0358) centre (67.9922, 27.7753) ccw
  arc A204 (67.7317, 27.3486) -> (67.5754, 27.3925) centre (67.5754, 27.0928) ccw
  line L188 (67.5754, 27.3925) -> (66.675, 27.3925)
  line L189 (66.675, 27.3925) -> (65.7746, 27.3925)
  arc A205 (65.7746, 27.3925) -> (65.6183, 27.3486) centre (65.7746, 27.0925) ccw
  arc A206 (64.9311, 28.0358) -> (65.6183, 27.3486) centre (65.3578, 27.7753) ccw
  arc A207 (64.9311, 28.0358) -> (64.975, 28.1921) centre (64.675, 28.1921) ccw
  line L190 (64.975, 28.1921) -> (64.975, 28.8925)
  line L191 (64.975, 28.8925) -> (64.975, 29.5929)
  arc A208 (64.975, 29.5929) -> (64.9311, 29.7492) centre (64.675, 29.5929) ccw
  arc A209 (65.6183, 30.4364) -> (64.9311, 29.7492) centre (65.3578, 30.0097) ccw
  arc A210 (65.6183, 30.4364) -> (65.7746, 30.3925) centre (65.7746, 30.6925) ccw
  line L192 (65.7746, 30.3925) -> (66.675, 30.3925)
  line L193 (66.675, 30.3925) -> (67.5754, 30.3925)
  arc A211 (67.5754, 30.3925) -> (67.7317, 30.4364) centre (67.5753, 30.6925) ccw
  arc A212 (68.4189, 29.7492) -> (67.7317, 30.4364) centre (67.9922, 30.0097) ccw
  arc A213 (68.4189, 29.7492) -> (68.375, 29.5929) centre (68.6751, 29.5928) ccw
  line L194 (68.375, 29.5929) -> (68.375, 28.8925)
  line L195 (68.375, 28.8925) -> (68.375, 28.1921)
  arc A214 (68.375, 28.1921) -> (68.4189, 28.0358) centre (68.675, 28.1922) ccw
  circle A215 centre (66.675, 23.8125) radius 1.9939
  circle A216 centre (61.595, 23.8125) radius 0.875
  circle A217 centre (52.705, 23.8125) radius 0.875
  circle A218 centre (89.535, 21.2725) radius 1.5
  circle A219 centre (83.185, 18.7325) radius 1.5
  circle A220 centre (70.485, 21.2725) radius 1.5
  circle A221 centre (64.135, 18.7325) radius 1.5
  circle A222 centre (51.435, 21.2725) radius 1.5
  circle A223 centre (43.18, 42.8625) radius 0.875
  circle A224 centre (38.1, 42.8625) radius 1.9939
  circle A225 centre (33.02, 42.8625) radius 0.875
  circle A226 centre (41.91, 40.3225) radius 1.5
  circle A227 centre (35.56, 37.7825) radius 1.5
  circle A228 centre (24.13, 42.8625) radius 0.875
  circle A229 centre (19.05, 42.8625) radius 1.9939
  circle A230 centre (13.97, 42.8625) radius 0.875
  circle A231 centre (22.86, 40.3225) radius 1.5
  circle A232 centre (16.51, 37.7825) radius 1.5
  circle A233 centre (5.08, 42.8625) radius 0.875
  circle A234 centre (0, 42.8625) radius 1.9939
  circle A235 centre (-5.08, 42.8625) radius 0.875
  circle A236 centre (3.81, 40.3225) radius 1.5
  circle A237 centre (-2.54, 37.7825) radius 1.5
  circle A238 centre (-13.97, 42.8625) radius 0.875
  circle A239 centre (-19.05, 42.8625) radius 1.9939
  circle A240 centre (-24.13, 42.8625) radius 0.875
  circle A241 centre (-15.24, 40.3225) radius 1.5
  circle A242 centre (-21.59, 37.7825) radius 1.5
  arc A243 (48.6817, 27.3486) -> (49.3689, 28.0358) centre (48.9422, 27.7753) ccw
  arc A244 (48.6817, 27.3486) -> (48.5254, 27.3925) centre (48.5254, 27.0928) ccw
  line L196 (48.5254, 27.3925) -> (47.625, 27.3925)
  line L197 (47.625, 27.3925) -> (46.7246, 27.3925)
  arc A245 (46.7246, 27.3925) -> (46.5683, 27.3486) centre (46.7246, 27.0925) ccw
  arc A246 (45.8811, 28.0358) -> (46.5683, 27.3486) centre (46.3078, 27.7753) ccw
  arc A247 (45.8811, 28.0358) -> (45.925, 28.1921) centre (45.625, 28.1921) ccw
  line L198 (45.925, 28.1921) -> (45.925, 28.8925)
  line L199 (45.925, 28.8925) -> (45.925, 29.5929)
  arc A248 (45.925, 29.5929) -> (45.8811, 29.7492) centre (45.625, 29.5929) ccw
  arc A249 (46.5683, 30.4364) -> (45.8811, 29.7492) centre (46.3078, 30.0097) ccw
  arc A250 (46.5683, 30.4364) -> (46.7246, 30.3925) centre (46.7246, 30.6925) ccw
  line L200 (46.7246, 30.3925) -> (47.625, 30.3925)
  line L201 (47.625, 30.3925) -> (48.5254, 30.3925)
  arc A251 (48.5254, 30.3925) -> (48.6817, 30.4364) centre (48.5253, 30.6925) ccw
  arc A252 (49.3689, 29.7492) -> (48.6817, 30.4364) centre (48.9422, 30.0097) ccw
  arc A253 (49.3689, 29.7492) -> (49.325, 29.5929) centre (49.6251, 29.5928) ccw
  line L202 (49.325, 29.5929) -> (49.325, 28.8925)
  line L203 (49.325, 28.8925) -> (49.325, 28.1921)
  arc A254 (49.325, 28.1921) -> (49.3689, 28.0358) centre (49.625, 28.1922) ccw
  circle A255 centre (47.625, 23.8125) radius 1.9939
  circle A256 centre (42.545, 23.8125) radius 0.875
  circle A257 centre (33.655, 23.8125) radius 0.875
  arc A258 (29.6317, 27.3486) -> (30.3189, 28.0358) centre (29.8922, 27.7753) ccw
  arc A259 (29.6317, 27.3486) -> (29.4754, 27.3925) centre (29.4754, 27.0928) ccw
  line L204 (29.4754, 27.3925) -> (28.575, 27.3925)
  line L205 (28.575, 27.3925) -> (27.6746, 27.3925)
  arc A260 (27.6746, 27.3925) -> (27.5183, 27.3486) centre (27.6746, 27.0925) ccw
  arc A261 (26.8311, 28.0358) -> (27.5183, 27.3486) centre (27.2578, 27.7753) ccw
  arc A262 (26.8311, 28.0358) -> (26.875, 28.1921) centre (26.575, 28.1921) ccw
  line L206 (26.875, 28.1921) -> (26.875, 28.8925)
  line L207 (26.875, 28.8925) -> (26.875, 29.5929)
  arc A263 (26.875, 29.5929) -> (26.8311, 29.7492) centre (26.575, 29.5929) ccw
  arc A264 (27.5183, 30.4364) -> (26.8311, 29.7492) centre (27.2578, 30.0097) ccw
  arc A265 (27.5183, 30.4364) -> (27.6746, 30.3925) centre (27.6746, 30.6925) ccw
  line L208 (27.6746, 30.3925) -> (28.575, 30.3925)
  line L209 (28.575, 30.3925) -> (29.4754, 30.3925)
  arc A266 (29.4754, 30.3925) -> (29.6317, 30.4364) centre (29.4753, 30.6925) ccw
  arc A267 (30.3189, 29.7492) -> (29.6317, 30.4364) centre (29.8922, 30.0097) ccw
  arc A268 (30.3189, 29.7492) -> (30.275, 29.5929) centre (30.5751, 29.5928) ccw
  line L210 (30.275, 29.5929) -> (30.275, 28.8925)
  line L211 (30.275, 28.8925) -> (30.275, 28.1921)
  arc A269 (30.275, 28.1921) -> (30.3189, 28.0358) centre (30.575, 28.1922) ccw
  circle A270 centre (28.575, 23.8125) radius 1.9939
  circle A271 centre (23.495, 23.8125) radius 0.875
  circle A272 centre (14.605, 23.8125) radius 0.875
  circle A273 centre (45.085, 18.7325) radius 1.5
  circle A274 centre (32.385, 21.2725) radius 1.5
  circle A275 centre (26.035, 18.7325) radius 1.5
  circle A276 centre (13.335, 21.2725) radius 1.5
  arc A277 (10.5817, 27.3486) -> (11.2689, 28.0358) centre (10.8422, 27.7753) ccw
  arc A278 (10.5817, 27.3486) -> (10.4254, 27.3925) centre (10.4254, 27.0928) ccw
  line L212 (10.4254, 27.3925) -> (9.525, 27.3925)
  line L213 (9.525, 27.3925) -> (8.6246, 27.3925)
  arc A279 (8.6246, 27.3925) -> (8.4683, 27.3486) centre (8.6246, 27.0925) ccw
  arc A280 (7.7811, 28.0358) -> (8.4683, 27.3486) centre (8.2078, 27.7753) ccw
  arc A281 (7.7811, 28.0358) -> (7.825, 28.1921) centre (7.525, 28.1921) ccw
  line L214 (7.825, 28.1921) -> (7.825, 28.8925)
  line L215 (7.825, 28.8925) -> (7.825, 29.5929)
  arc A282 (7.825, 29.5929) -> (7.7811, 29.7492) centre (7.525, 29.5929) ccw
  arc A283 (8.4683, 30.4364) -> (7.7811, 29.7492) centre (8.2078, 30.0097) ccw
  arc A284 (8.4683, 30.4364) -> (8.6246, 30.3925) centre (8.6246, 30.6925) ccw
  line L216 (8.6246, 30.3925) -> (9.525, 30.3925)
  line L217 (9.525, 30.3925) -> (10.4254, 30.3925)
  arc A285 (10.4254, 30.3925) -> (10.5817, 30.4364) centre (10.4253, 30.6925) ccw
  arc A286 (11.2689, 29.7492) -> (10.5817, 30.4364) centre (10.8422, 30.0097) ccw
  arc A287 (11.2689, 29.7492) -> (11.225, 29.5929) centre (11.5251, 29.5928) ccw
  line L218 (11.225, 29.5929) -> (11.225, 28.8925)
  line L219 (11.225, 28.8925) -> (11.225, 28.1921)
  arc A288 (11.225, 28.1921) -> (11.2689, 28.0358) centre (11.525, 28.1922) ccw
  circle A289 centre (9.525, 23.8125) radius 1.9939
  circle A290 centre (4.445, 23.8125) radius 0.875
  circle A291 centre (-4.445, 23.8125) radius 0.875
  arc A292 (-11.2689, 28.0358) -> (-10.5817, 27.3486) centre (-10.8422, 27.7753) ccw
  arc A293 (-11.2689, 28.0358) -> (-11.225, 28.1921) centre (-11.525, 28.1921) ccw
  line L220 (-11.225, 28.1921) -> (-11.225, 28.8925)
  line L221 (-11.225, 28.8925) -> (-11.225, 29.5929)
  arc A294 (-11.225, 29.5929) -> (-11.2689, 29.7492) centre (-11.525, 29.5929) ccw
  arc A295 (-10.5817, 30.4364) -> (-11.2689, 29.7492) centre (-10.8422, 30.0097) ccw
  arc A296 (-10.5817, 30.4364) -> (-10.4254, 30.3925) centre (-10.4254, 30.6925) ccw
  line L222 (-10.4254, 30.3925) -> (-9.525, 30.3925)
  line L223 (-9.525, 30.3925) -> (-8.6246, 30.3925)
  arc A297 (-8.6246, 30.3925) -> (-8.4683, 30.4364) centre (-8.6247, 30.6925) ccw
  arc A298 (-7.7811, 29.7492) -> (-8.4683, 30.4364) centre (-8.2078, 30.0097) ccw
  arc A299 (-7.7811, 29.7492) -> (-7.825, 29.5929) centre (-7.5249, 29.5928) ccw
  line L224 (-7.825, 29.5929) -> (-7.825, 28.8925)
  line L225 (-7.825, 28.8925) -> (-7.825, 28.1921)
  arc A300 (-7.825, 28.1921) -> (-7.7811, 28.0358) centre (-7.525, 28.1922) ccw
  arc A301 (-8.4683, 27.3486) -> (-7.7811, 28.0358) centre (-8.2078, 27.7753) ccw
  arc A302 (-8.4683, 27.3486) -> (-8.6246, 27.3925) centre (-8.6246, 27.0928) ccw
  line L226 (-8.6246, 27.3925) -> (-9.525, 27.3925)
  line L227 (-9.525, 27.3925) -> (-10.4254, 27.3925)
  arc A303 (-10.4254, 27.3925) -> (-10.5817, 27.3486) centre (-10.4254, 27.0925) ccw
  arc A304 (-30.3189, 28.0358) -> (-29.6317, 27.3486) centre (-29.8922, 27.7753) ccw
  arc A305 (-30.3189, 28.0358) -> (-30.275, 28.1921) centre (-30.575, 28.1921) ccw
  line L228 (-30.275, 28.1921) -> (-30.275, 28.8925)
  line L229 (-30.275, 28.8925) -> (-30.275, 29.5929)
  arc A306 (-30.275, 29.5929) -> (-30.3189, 29.7492) centre (-30.575, 29.5929) ccw
  arc A307 (-29.6317, 30.4364) -> (-30.3189, 29.7492) centre (-29.8922, 30.0097) ccw
  arc A308 (-29.6317, 30.4364) -> (-29.4754, 30.3925) centre (-29.4754, 30.6925) ccw
  line L230 (-29.4754, 30.3925) -> (-28.575, 30.3925)
  line L231 (-28.575, 30.3925) -> (-27.6746, 30.3925)
  arc A309 (-27.6746, 30.3925) -> (-27.5183, 30.4364) centre (-27.6747, 30.6925) ccw
  arc A310 (-26.8311, 29.7492) -> (-27.5183, 30.4364) centre (-27.2578, 30.0097) ccw
  arc A311 (-26.8311, 29.7492) -> (-26.875, 29.5929) centre (-26.5749, 29.5928) ccw
  line L232 (-26.875, 29.5929) -> (-26.875, 28.8925)
  line L233 (-26.875, 28.8925) -> (-26.875, 28.1921)
  arc A312 (-26.875, 28.1921) -> (-26.8311, 28.0358) centre (-26.575, 28.1922) ccw
  arc A313 (-27.5183, 27.3486) -> (-26.8311, 28.0358) centre (-27.2578, 27.7753) ccw
  arc A314 (-27.5183, 27.3486) -> (-27.6746, 27.3925) centre (-27.6746, 27.0928) ccw
  line L234 (-27.6746, 27.3925) -> (-28.575, 27.3925)
  line L235 (-28.575, 27.3925) -> (-29.4754, 27.3925)
  arc A315 (-29.4754, 27.3925) -> (-29.6317, 27.3486) centre (-29.4754, 27.0925) ccw
  circle A316 centre (-9.525, 23.8125) radius 1.9939
  circle A317 centre (-14.605, 23.8125) radius 0.875
  circle A318 centre (-23.495, 23.8125) radius 0.875
  circle A319 centre (-28.575, 23.8125) radius 1.9939
  circle A320 centre (6.985, 18.7325) radius 1.5
  circle A321 centre (-5.715, 21.2725) radius 1.5
  circle A322 centre (-12.065, 18.7325) radius 1.5
  circle A323 centre (-24.765, 21.2725) radius 1.5
  circle A324 centre (-50.0063, 76.2) radius 1.1
  circle A325 centre (-66.3575, 61.9125) radius 0.875
  arc A326 (-73.1814, 66.1358) -> (-72.4942, 65.4486) centre (-72.7547, 65.8753) ccw
  arc A327 (-73.1814, 66.1358) -> (-73.1375, 66.2921) centre (-73.4375, 66.2921) ccw
  line L236 (-73.1375, 66.2921) -> (-73.1375, 66.9925)
  line L237 (-73.1375, 66.9925) -> (-73.1375, 67.6929)
  arc A328 (-73.1375, 67.6929) -> (-73.1814, 67.8492) centre (-73.4375, 67.6929) ccw
  arc A329 (-72.4942, 68.5364) -> (-73.1814, 67.8492) centre (-72.7547, 68.1097) ccw
  arc A330 (-72.4942, 68.5364) -> (-72.3379, 68.4925) centre (-72.3379, 68.7925) ccw
  line L238 (-72.3379, 68.4925) -> (-71.4375, 68.4925)
  line L239 (-71.4375, 68.4925) -> (-70.5371, 68.4925)
  arc A331 (-70.5371, 68.4925) -> (-70.3808, 68.5364) centre (-70.5372, 68.7925) ccw
  arc A332 (-69.6936, 67.8492) -> (-70.3808, 68.5364) centre (-70.1203, 68.1097) ccw
  arc A333 (-69.6936, 67.8492) -> (-69.7375, 67.6929) centre (-69.4374, 67.6928) ccw
  line L240 (-69.7375, 67.6929) -> (-69.7375, 66.9925)
  line L241 (-69.7375, 66.9925) -> (-69.7375, 66.2921)
  arc A334 (-69.7375, 66.2921) -> (-69.6936, 66.1358) centre (-69.4375, 66.2922) ccw
  arc A335 (-70.3808, 65.4486) -> (-69.6936, 66.1358) centre (-70.1203, 65.8753) ccw
  arc A336 (-70.3808, 65.4486) -> (-70.5371, 65.4925) centre (-70.5371, 65.1928) ccw
  line L242 (-70.5371, 65.4925) -> (-71.4375, 65.4925)
  line L243 (-71.4375, 65.4925) -> (-72.3379, 65.4925)
  arc A337 (-72.3379, 65.4925) -> (-72.4942, 65.4486) centre (-72.3379, 65.1925) ccw
  circle A338 centre (-71.4375, 61.9125) radius 1.9939
  circle A339 centre (-76.5175, 61.9125) radius 0.875
  circle A340 centre (-85.4075, 61.9125) radius 0.875
  arc A341 (-92.2314, 66.1358) -> (-91.5442, 65.4486) centre (-91.8047, 65.8753) ccw
  arc A342 (-92.2314, 66.1358) -> (-92.1875, 66.2921) centre (-92.4875, 66.2921) ccw
  line L244 (-92.1875, 66.2921) -> (-92.1875, 66.9925)
  line L245 (-92.1875, 66.9925) -> (-92.1875, 67.6929)
  arc A343 (-92.1875, 67.6929) -> (-92.2314, 67.8492) centre (-92.4875, 67.6929) ccw
  arc A344 (-91.5442, 68.5364) -> (-92.2314, 67.8492) centre (-91.8047, 68.1097) ccw
  arc A345 (-91.5442, 68.5364) -> (-91.3879, 68.4925) centre (-91.3879, 68.7925) ccw
  line L246 (-91.3879, 68.4925) -> (-90.4875, 68.4925)
  line L247 (-90.4875, 68.4925) -> (-89.5871, 68.4925)
  arc A346 (-89.5871, 68.4925) -> (-89.4308, 68.5364) centre (-89.5872, 68.7925) ccw
  arc A347 (-88.7436, 67.8492) -> (-89.4308, 68.5364) centre (-89.1703, 68.1097) ccw
  arc A348 (-88.7436, 67.8492) -> (-88.7875, 67.6929) centre (-88.4874, 67.6928) ccw
  line L248 (-88.7875, 67.6929) -> (-88.7875, 66.9925)
  line L249 (-88.7875, 66.9925) -> (-88.7875, 66.2921)
  arc A349 (-88.7875, 66.2921) -> (-88.7436, 66.1358) centre (-88.4875, 66.2922) ccw
  arc A350 (-89.4308, 65.4486) -> (-88.7436, 66.1358) centre (-89.1703, 65.8753) ccw
  arc A351 (-89.4308, 65.4486) -> (-89.5871, 65.4925) centre (-89.5871, 65.1928) ccw
  line L250 (-89.5871, 65.4925) -> (-90.4875, 65.4925)
  line L251 (-90.4875, 65.4925) -> (-91.3879, 65.4925)
  arc A352 (-91.3879, 65.4925) -> (-91.5442, 65.4486) centre (-91.3879, 65.1925) ccw
  circle A353 centre (-90.4875, 61.9125) radius 1.9939
  circle A354 centre (-95.5675, 61.9125) radius 0.875
  circle A355 centre (-104.4575, 61.9125) radius 0.875
  circle A356 centre (-67.6275, 59.3725) radius 1.5
  arc A357 (-39.8439, 47.0858) -> (-39.1567, 46.3986) centre (-39.4172, 46.8253) ccw
  arc A358 (-39.8439, 47.0858) -> (-39.8, 47.2421) centre (-40.1, 47.2421) ccw
  line L252 (-39.8, 47.2421) -> (-39.8, 47.9425)
  line L253 (-39.8, 47.9425) -> (-39.8, 48.6429)
  arc A359 (-39.8, 48.6429) -> (-39.8439, 48.7992) centre (-40.1, 48.6429) ccw
  arc A360 (-39.1567, 49.4864) -> (-39.8439, 48.7992) centre (-39.4172, 49.0597) ccw
  arc A361 (-39.1567, 49.4864) -> (-39.0004, 49.4425) centre (-39.0004, 49.7425) ccw
  line L254 (-39.0004, 49.4425) -> (-38.1, 49.4425)
  line L255 (-38.1, 49.4425) -> (-37.1996, 49.4425)
  arc A362 (-37.1996, 49.4425) -> (-37.0433, 49.4864) centre (-37.1997, 49.7425) ccw
  arc A363 (-36.3561, 48.7992) -> (-37.0433, 49.4864) centre (-36.7828, 49.0597) ccw
  arc A364 (-36.3561, 48.7992) -> (-36.4, 48.6429) centre (-36.0999, 48.6428) ccw
  line L256 (-36.4, 48.6429) -> (-36.4, 47.9425)
  line L257 (-36.4, 47.9425) -> (-36.4, 47.2421)
  arc A365 (-36.4, 47.2421) -> (-36.3561, 47.0858) centre (-36.1, 47.2422) ccw
  arc A366 (-37.0433, 46.3986) -> (-36.3561, 47.0858) centre (-36.7828, 46.8253) ccw
  arc A367 (-37.0433, 46.3986) -> (-37.1996, 46.4425) centre (-37.1996, 46.1428) ccw
  line L258 (-37.1996, 46.4425) -> (-38.1, 46.4425)
  line L259 (-38.1, 46.4425) -> (-39.0004, 46.4425)
  arc A368 (-39.0004, 46.4425) -> (-39.1567, 46.3986) centre (-39.0004, 46.1425) ccw
  arc A369 (-58.8939, 47.0858) -> (-58.2067, 46.3986) centre (-58.4672, 46.8253) ccw
  arc A370 (-58.8939, 47.0858) -> (-58.85, 47.2421) centre (-59.15, 47.2421) ccw
  line L260 (-58.85, 47.2421) -> (-58.85, 47.9425)
  line L261 (-58.85, 47.9425) -> (-58.85, 48.6429)
  arc A371 (-58.85, 48.6429) -> (-58.8939, 48.7992) centre (-59.15, 48.6429) ccw
  arc A372 (-58.2067, 49.4864) -> (-58.8939, 48.7992) centre (-58.4672, 49.0597) ccw
  arc A373 (-58.2067, 49.4864) -> (-58.0504, 49.4425) centre (-58.0504, 49.7425) ccw
  line L262 (-58.0504, 49.4425) -> (-57.15, 49.4425)
  line L263 (-57.15, 49.4425) -> (-56.2496, 49.4425)
  arc A374 (-56.2496, 49.4425) -> (-56.0933, 49.4864) centre (-56.2497, 49.7425) ccw
  arc A375 (-55.4061, 48.7992) -> (-56.0933, 49.4864) centre (-55.8328, 49.0597) ccw
  arc A376 (-55.4061, 48.7992) -> (-55.45, 48.6429) centre (-55.1499, 48.6428) ccw
  line L264 (-55.45, 48.6429) -> (-55.45, 47.9425)
  line L265 (-55.45, 47.9425) -> (-55.45, 47.2421)
  arc A377 (-55.45, 47.2421) -> (-55.4061, 47.0858) centre (-55.15, 47.2422) ccw
  arc A378 (-56.0933, 46.3986) -> (-55.4061, 47.0858) centre (-55.8328, 46.8253) ccw
  arc A379 (-56.0933, 46.3986) -> (-56.2496, 46.4425) centre (-56.2496, 46.1428) ccw
  line L266 (-56.2496, 46.4425) -> (-57.15, 46.4425)
  line L267 (-57.15, 46.4425) -> (-58.0504, 46.4425)
  arc A380 (-58.0504, 46.4425) -> (-58.2067, 46.3986) centre (-58.0504, 46.1425) ccw
  circle A381 centre (-86.6775, 59.3725) radius 1.5
  circle A382 centre (-73.9775, 56.8325) radius 1.5
  circle A383 centre (-105.7275, 59.3725) radius 1.5
  circle A384 centre (-93.0275, 56.8325) radius 1.5
  arc A385 (-77.9439, 47.0858) -> (-77.2567, 46.3986) centre (-77.5172, 46.8253) ccw
  arc A386 (-77.9439, 47.0858) -> (-77.9, 47.2421) centre (-78.2, 47.2421) ccw
  line L268 (-77.9, 47.2421) -> (-77.9, 47.9425)
  line L269 (-77.9, 47.9425) -> (-77.9, 48.6429)
  arc A387 (-77.9, 48.6429) -> (-77.9439, 48.7992) centre (-78.2, 48.6429) ccw
  arc A388 (-77.2567, 49.4864) -> (-77.9439, 48.7992) centre (-77.5172, 49.0597) ccw
  arc A389 (-77.2567, 49.4864) -> (-77.1004, 49.4425) centre (-77.1004, 49.7425) ccw
  line L270 (-77.1004, 49.4425) -> (-76.2, 49.4425)
  line L271 (-76.2, 49.4425) -> (-75.2996, 49.4425)
  arc A390 (-75.2996, 49.4425) -> (-75.1433, 49.4864) centre (-75.2997, 49.7425) ccw
  arc A391 (-74.4561, 48.7992) -> (-75.1433, 49.4864) centre (-74.8828, 49.0597) ccw
  arc A392 (-74.4561, 48.7992) -> (-74.5, 48.6429) centre (-74.1999, 48.6428) ccw
  line L272 (-74.5, 48.6429) -> (-74.5, 47.9425)
  line L273 (-74.5, 47.9425) -> (-74.5, 47.2421)
  arc A393 (-74.5, 47.2421) -> (-74.4561, 47.0858) centre (-74.2, 47.2422) ccw
  arc A394 (-75.1433, 46.3986) -> (-74.4561, 47.0858) centre (-74.8828, 46.8253) ccw
  arc A395 (-75.1433, 46.3986) -> (-75.2996, 46.4425) centre (-75.2996, 46.1428) ccw
  line L274 (-75.2996, 46.4425) -> (-76.2, 46.4425)
  line L275 (-76.2, 46.4425) -> (-77.1004, 46.4425)
  arc A396 (-77.1004, 46.4425) -> (-77.2567, 46.3986) centre (-77.1004, 46.1425) ccw
  arc A397 (-96.9939, 47.0858) -> (-96.3067, 46.3986) centre (-96.5672, 46.8253) ccw
  arc A398 (-96.9939, 47.0858) -> (-96.95, 47.2421) centre (-97.25, 47.2421) ccw
  line L276 (-96.95, 47.2421) -> (-96.95, 47.9425)
  line L277 (-96.95, 47.9425) -> (-96.95, 48.6429)
  arc A399 (-96.95, 48.6429) -> (-96.9939, 48.7992) centre (-97.25, 48.6429) ccw
  arc A400 (-96.3067, 49.4864) -> (-96.9939, 48.7992) centre (-96.5672, 49.0597) ccw
  arc A401 (-96.3067, 49.4864) -> (-96.1504, 49.4425) centre (-96.1504, 49.7425) ccw
  line L278 (-96.1504, 49.4425) -> (-95.25, 49.4425)
  line L279 (-95.25, 49.4425) -> (-94.3496, 49.4425)
  arc A402 (-94.3496, 49.4425) -> (-94.1933, 49.4864) centre (-94.3497, 49.7425) ccw
  arc A403 (-93.5061, 48.7992) -> (-94.1933, 49.4864) centre (-93.9328, 49.0597) ccw
  arc A404 (-93.5061, 48.7992) -> (-93.55, 48.6429) centre (-93.2499, 48.6428) ccw
  line L280 (-93.55, 48.6429) -> (-93.55, 47.9425)
  line L281 (-93.55, 47.9425) -> (-93.55, 47.2421)
  arc A405 (-93.55, 47.2421) -> (-93.5061, 47.0858) centre (-93.25, 47.2422) ccw
  arc A406 (-94.1933, 46.3986) -> (-93.5061, 47.0858) centre (-93.9328, 46.8253) ccw
  arc A407 (-94.1933, 46.3986) -> (-94.3496, 46.4425) centre (-94.3496, 46.1428) ccw
  line L282 (-94.3496, 46.4425) -> (-95.25, 46.4425)
  line L283 (-95.25, 46.4425) -> (-96.1504, 46.4425)
  arc A408 (-96.1504, 46.4425) -> (-96.3067, 46.3986) centre (-96.1504, 46.1425) ccw
  arc A409 (-135.0939, 70.8983) -> (-134.4067, 70.2111) centre (-134.6672, 70.6378) ccw
  arc A410 (-135.0939, 70.8983) -> (-135.05, 71.0546) centre (-135.35, 71.0546) ccw
  line L284 (-135.05, 71.0546) -> (-135.05, 71.755)
  line L285 (-135.05, 71.755) -> (-135.05, 72.4554)
  arc A411 (-135.05, 72.4554) -> (-135.0939, 72.6117) centre (-135.35, 72.4554) ccw
  arc A412 (-134.4067, 73.2989) -> (-135.0939, 72.6117) centre (-134.6672, 72.8722) ccw
  arc A413 (-134.4067, 73.2989) -> (-134.2504, 73.255) centre (-134.2504, 73.555) ccw
  line L286 (-134.2504, 73.255) -> (-133.35, 73.255)
  line L287 (-133.35, 73.255) -> (-132.4496, 73.255)
  arc A414 (-132.4496, 73.255) -> (-132.2933, 73.2989) centre (-132.4497, 73.555) ccw
  arc A415 (-131.6061, 72.6117) -> (-132.2933, 73.2989) centre (-132.0328, 72.8722) ccw
  arc A416 (-131.6061, 72.6117) -> (-131.65, 72.4554) centre (-131.3499, 72.4553) ccw
  line L288 (-131.65, 72.4554) -> (-131.65, 71.755)
  line L289 (-131.65, 71.755) -> (-131.65, 71.0546)
  arc A417 (-131.65, 71.0546) -> (-131.6061, 70.8983) centre (-131.35, 71.0547) ccw
  arc A418 (-132.2933, 70.2111) -> (-131.6061, 70.8983) centre (-132.0328, 70.6378) ccw
  arc A419 (-132.2933, 70.2111) -> (-132.4496, 70.255) centre (-132.4496, 69.9553) ccw
  line L290 (-132.4496, 70.255) -> (-133.35, 70.255)
  line L291 (-133.35, 70.255) -> (-134.2504, 70.255)
  arc A420 (-134.2504, 70.255) -> (-134.4067, 70.2111) centre (-134.2504, 69.955) ccw
  arc A421 (-111.2814, 66.1358) -> (-110.5942, 65.4486) centre (-110.8547, 65.8753) ccw
  arc A422 (-111.2814, 66.1358) -> (-111.2375, 66.2921) centre (-111.5375, 66.2921) ccw
  line L292 (-111.2375, 66.2921) -> (-111.2375, 66.9925)
  line L293 (-111.2375, 66.9925) -> (-111.2375, 67.6929)
  arc A423 (-111.2375, 67.6929) -> (-111.2814, 67.8492) centre (-111.5375, 67.6929) ccw
  arc A424 (-110.5942, 68.5364) -> (-111.2814, 67.8492) centre (-110.8547, 68.1097) ccw
  arc A425 (-110.5942, 68.5364) -> (-110.4379, 68.4925) centre (-110.4379, 68.7925) ccw
  line L294 (-110.4379, 68.4925) -> (-109.5375, 68.4925)
  line L295 (-109.5375, 68.4925) -> (-108.6371, 68.4925)
  arc A426 (-108.6371, 68.4925) -> (-108.4808, 68.5364) centre (-108.6372, 68.7925) ccw
  arc A427 (-107.7936, 67.8492) -> (-108.4808, 68.5364) centre (-108.2203, 68.1097) ccw
  arc A428 (-107.7936, 67.8492) -> (-107.8375, 67.6929) centre (-107.5374, 67.6928) ccw
  line L296 (-107.8375, 67.6929) -> (-107.8375, 66.9925)